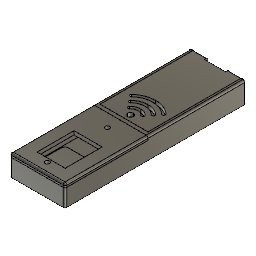
sensor_case (Autodesk Fusion 360 design; units mm, degrees)
Autodesk Fusion 360 part; units mm, degrees
sketch "MainBottom" plane through (0, 0, 0) normal (0, 0, 1) x (1, 0, 0)
  line L0 (0, 0) -> (30, 0)
  line L1 (30, 0) -> (30, 53.3)
  line L2 (30, 53.3) -> (0, 53.3)
  line L3 (0, 53.3) -> (0, 0)
  dimension "d3" = 53.3
  dimension "d4" = 30
  constraint horizontal L0
  constraint vertical L1
  constraint horizontal L2
  constraint vertical L3
  constraint coincident L0.start L3.end
  measures "d3" distance of L0.end L1.end
  measures "d4" distance of L1.end L2.end
extrude "Extrude1" add sketch "MainBottom" along normal blind 2 makes body 1
sketch "MainRight" plane through (30, 0, 0) normal (1, 0, 0) x (0, 1, 0)
  line L0 (0, 0) -> (53.3, 0)
  line L1 (53.3, 0) -> (53.3, 2)
  line L2 (53.3, 2) -> (0, 2)
  line L3 (0, 2) -> (0, 0)
  line L4 (53.3, 2) -> (0, 2)
  line L5 (0, 2) -> (0, 11.5)
  line L6 (0, 11.5) -> (53.3, 11.5)
  line L7 (53.3, 11.5) -> (53.3, 2)
  dimension "d9" = 9.5
  constraint horizontal L4
  constraint vertical L5
  constraint horizontal L6
  constraint vertical L7
  constraint coincident L1.end L2.start
  constraint coincident L2.end L3.start
  measures "d9" distance of L1.end L6.end
extrude "Extrude2" add sketch "MainRight" against normal blind 2 contours L2 L4 L5 L6 L7 bodies 1
sketch "MainLeft" plane through (0, 0, 0) normal (-1, 0, 0) x (0, -1, 0)
  line L0 (-53.3, 0) -> (0, 0)
  line L1 (0, 0) -> (0, 2)
  line L2 (0, 2) -> (-53.3, 2)
  line L3 (-53.3, 2) -> (-53.3, 0)
  line L4 (0, 2) -> (-53.3, 2)
  line L5 (-53.3, 2) -> (-53.3, 11.5)
  line L6 (-53.3, 11.5) -> (0, 11.5)
  line L7 (0, 11.5) -> (0, 2)
  dimension "d12" = 9.5
  constraint horizontal L4
  constraint vertical L5
  constraint horizontal L6
  constraint vertical L7
  constraint coincident L1.end L2.start
  constraint coincident L2.end L3.start
  measures "d12" distance of L1.end L6.end
extrude "Extrude3" add sketch "MainLeft" against normal blind 2 contours L2 L4 L5 L6 L7 bodies 1
sketch "MainFront" plane through (0, 0, 0) normal (0, -1, 0) x (1, 0, 0)
  line L0 (0, 0) -> (30, 0)
  line L1 (30, 0) -> (30, 11.5)
  line L2 (30, 11.5) -> (28, 11.5)
  line L3 (28, 11.5) -> (28, 2)
  line L4 (28, 2) -> (2, 2)
  line L5 (2, 2) -> (2, 11.5)
  line L6 (2, 11.5) -> (0, 11.5)
  line L7 (0, 11.5) -> (0, 0)
  line L8 (2, 2) -> (28, 2)
  line L9 (28, 2) -> (28, 11.5)
  line L10 (28, 11.5) -> (2, 11.5)
  line L11 (2, 11.5) -> (2, 2)
  dimension "d367" = 9.5
  constraint horizontal L8
  constraint vertical L9
  constraint horizontal L10
  constraint vertical L11
  constraint coincident L4.end L5.start
  constraint coincident L3 L2.end
  measures "d367" distance of L3.end L2.end
extrude "Extrude4" add sketch "MainFront" against normal blind 2 contours L3 L4 L5 L8 L9 L10 L11 bodies 1
sketch "MainBack" plane through (0, 53.3, 0) normal (0, 1, 0) x (-1, 0, 0)
  line L0 (-30, 0) -> (0, 0)
  line L1 (0, 0) -> (0, 11.5)
  line L2 (0, 11.5) -> (-2, 11.5)
  line L3 (-2, 11.5) -> (-2, 2)
  line L4 (-2, 2) -> (-28, 2)
  line L5 (-28, 2) -> (-28, 11.5)
  line L6 (-28, 11.5) -> (-30, 11.5)
  line L7 (-30, 11.5) -> (-30, 0)
  line L8 (-28, 2) -> (-2, 2)
  line L9 (-2, 2) -> (-2, 11.5)
  line L10 (-2, 11.5) -> (-28, 11.5)
  line L11 (-28, 11.5) -> (-28, 2)
  constraint horizontal L8
  constraint vertical L9
  constraint horizontal L10
  constraint vertical L11
  constraint coincident L2.end L3.start
  constraint coincident L4.end L5.start
extrude "Extrude5" add sketch "MainBack" against normal blind 2 contours L3 L4 L5 L8 L9 L10 L11 bodies 1
sketch "DeviceSupportBack" plane through (0, 0, 2) normal (0, 0, 1) x (-1, 0, 0)
  line L0 (-28, -51.3) -> (-2, -51.3)
  line L1 (-2, -51.3) -> (-2, -2)
  line L2 (-2, -2) -> (-28, -2)
  line L3 (-28, -2) -> (-28, -51.3)
  line L4 (-28, -51.3) -> (-2, -51.3)
  line L5 (-2, -51.3) -> (-2, -46.3)
  line L6 (-2, -46.3) -> (-28, -46.3)
  line L7 (-28, -46.3) -> (-28, -51.3)
  dimension "d21" = 5
  constraint horizontal L4
  constraint vertical L5
  constraint horizontal L6
  constraint vertical L7
  constraint coincident L1 L5.end
  constraint coincident L0.start L3.end
  measures "d21" distance of L0.start L6.end
sketch "SensorBottom" plane through (0, 0, 0) normal (0, 0, -1) x (1, 0, 0)
  line L0 (0, 0) -> (0, -53.3)
  line L1 (0, -53.3) -> (30, -53.3)
  line L2 (30, -53.3) -> (30, 0)
  line L3 (30, 0) -> (0, 0)
  line L4 (0, 0) -> (30, 0)
  line L5 (30, 0) -> (30, 45)
  line L6 (30, 45) -> (0, 45)
  line L7 (0, 45) -> (0, 0)
  dimension "d144" = 30
  dimension "d145" = 45
  constraint horizontal L4
  constraint vertical L5
  constraint horizontal L6
  constraint vertical L7
  constraint midpoint L3 L4
  measures "d144" distance of L5.end L6.end
  measures "d145" distance of L2.end L5.end
extrude "Extrude17" add sketch "SensorBottom" against normal blind 2 contours L3 L4 L5 L6 L7 bodies 1
extrude "Extrude6" add sketch "DeviceSupportBack" along normal blind 3 contours L0 L1 L3 L4 L5 L6 L7 bodies 1
sketch "DeviceSupportFront" plane through (0, 0, 2) normal (0, 0, 1) x (-1, 0, 0)
  line L0 (-28, -46.3) -> (-2, -46.3)
  line L1 (-2, -46.3) -> (-2, -2)
  line L2 (-2, -2) -> (-28, -2)
  line L3 (-28, -2) -> (-28, -46.3)
  line L4 (-2, -2) -> (-28, -2)
  line L5 (-28, -2) -> (-28, -7)
  line L6 (-28, -7) -> (-2, -7)
  line L7 (-2, -7) -> (-2, -2)
  dimension "d24" = 5
  constraint horizontal L4
  constraint vertical L5
  constraint horizontal L6
  constraint vertical L7
  constraint coincident L3 L5.end
  constraint coincident L1.end L2.start
  measures "d24" distance of L1.end L6.end
extrude "Extrude7" add sketch "DeviceSupportFront" along normal blind 3 contours L1 L2 L3 L4 L5 L6 L7 bodies 1
sketch "DevicePosts" plane through (0, 0, 5) normal (0, 0, 1) x (-1, 0, 0)
  line L0 (-2, -46.3) -> (-28, -46.3)
  circle A0 centre (-25.256, -48.0042) radius 0.95
  line L1 (-2.25, -51) -> (-12.25, -51)
  circle A1 centre (-5.256, -48.0042) radius 0.95
  line L2 (-15.256, -51.0085) -> (-15.256, -2) construction
  line L3 (-15.256, -48.0042) -> (-25.256, -48.0042) construction
  line L4 (-28, -2) -> (-2, -2) construction
  line L5 (-15.256, -26.5042) -> (-15.256, -48.0042) construction
  line L6 (-15.256, -48.0042) -> (-5.256, -48.0042) construction
  line L7 (-15.256, -26.5042) -> (-15.256, -5.0042) construction
  circle A2 centre (-5.256, -5.0042) radius 0.95
  circle A3 centre (-25.256, -5.0042) radius 0.95
  line L8 (-15.256, -5.0042) -> (-5.256, -5.0042) construction
  line L9 (-15.256, -5.0042) -> (-25.256, -5.0042) construction
  line L10 (-28, -46.3) -> (-28, -51.3)
  line L11 (-28, -51.3) -> (-2, -51.3)
  line L12 (-2, -51.3) -> (-2, -46.3)
  dimension "d31" = 1.9
  dimension "d38" = 10
  dimension "d40" = 1.9
  dimension "d59" = 10
  dimension "d60" = 21.5
  dimension "d61" = 10
  dimension "d63" = 1.9
  dimension "d64" = 1.9
  dimension "d65" = 10
  dimension "d67" = 10
  dimension "d68" = 21.5
  constraint vertical L2
  constraint coincident L2 L3.start
  constraint coincident A0.centre L3.end
  constraint perpendicular L2 L3
  constraint coincident L2.end L4
  constraint midpoint L2 L5.start
  constraint parallel L2 L5
  constraint coincident L3.start L5.end
  constraint coincident A1.centre L6.end
  constraint perpendicular L2 L6
  constraint parallel L2 L7
  constraint coincident A2.centre L8.end
  constraint perpendicular L2 L8
  constraint coincident A3.centre L9.end
  constraint perpendicular L7 L9
  measures "d31" diameter of A0
  measures "d38" distance of L1.start L1.end
  measures "d40" diameter of A1
  measures "d59" horizontal distance of L3.start A0.centre
  measures "d60" vertical distance of L5.start L3.start
  measures "d61" distance of L3.start A1.centre
  measures "d63" diameter of A2
  measures "d64" diameter of A3
  measures "d65" horizontal distance of L7.end A2.centre
  measures "d67" horizontal distance of L7.end A3.centre
  measures "d68" distance of L5.start L7.end
extrude "Extrude8" cut sketch "DevicePosts" against normal blind 3 contours A0 | A1 | A2 | A3 bodies 1
sketch "USBPlugOpening" plane through (0, 53.3, 0) normal (0, 1, 0) x (-1, 0, 0)
  line L0 (-30, 0) -> (0, 0)
  line L1 (-15, 7.05) -> (-15, 0) construction
  line L2 (-20.75, 11.175) -> (-9.25, 11.175)
  line L3 (-9.25, 11.175) -> (-9.25, 2.925)
  line L4 (-9.25, 2.925) -> (-20.75, 2.925)
  line L5 (-20.75, 2.925) -> (-20.75, 11.175)
  line L6 (-20.75, 11.175) -> (-9.25, 11.175)
  line L7 (-9.25, 11.175) -> (-9.25, 16.175)
  line L8 (-9.25, 16.175) -> (-20.75, 16.175)
  line L9 (-20.75, 16.175) -> (-20.75, 11.175)
  line L10 (-20.75, 7.05) -> (-9.25, 7.05) construction
  dimension "d392" = 7.05
  dimension "d398" = 11.5
  dimension "d399" = 8.25
  dimension "d400" = 5
  constraint midpoint L0 L1.end
  constraint perpendicular L0 L1
  constraint horizontal L2
  constraint vertical L3
  constraint horizontal L4
  constraint vertical L5
  constraint horizontal L6
  constraint vertical L7
  constraint horizontal L8
  constraint vertical L9
  constraint coincident L2.start L5.end
  constraint coincident L2.end L3.start
  constraint midpoint L5 L10.start
  constraint midpoint L3 L10.end
  constraint midpoint L1.start L10
  measures "d392" distance of L1.start L1.end
  measures "d398" distance of L2.start L2.end
  measures "d399" distance of L2.start L4.end
  measures "d400" distance of L2.start L8.end
ref_plane "WorkPlane1" through (15, 26.65, 5.75) normal (1, 0, 0) x (0, 1, 0)
ref_plane "WorkPlane2" through (15, 26.65, 5.75) normal (0, -1, 0) x (1, 0, 0)
sketch "Lid" plane through (0, 53.3, 0) normal (0, 1, 0) x (-1, 0, 0)
  line L0 (-30, 0) -> (0, 0)
  line L1 (0, 0) -> (0, 11.5)
  line L2 (-30, 11.5) -> (-30, 0)
  line L3 (0, 11.5) -> (-2, 11.5)
  line L4 (-30, 11.5) -> (-28, 11.5) construction
  line L5 (-28, 11.5) -> (-2, 11.5)
  line L6 (-28, 11.5) -> (-29, 9.5)
  line L7 (-29, 9.5) -> (-1, 9.5)
  line L8 (-1, 9.5) -> (-2, 11.5)
  line L9 (-15, 11.5) -> (-15, 9.5) construction
  line L10 (-1, 9.5) -> (0, 9.5) construction
  dimension "d119" = 2
  dimension "d120" = 2
  dimension "d121" = 2
  dimension "d122" = 1
  constraint coincident L1.end L3.start
  constraint perpendicular L1 L3
  constraint coincident L2.start L4.start
  constraint perpendicular L2 L4
  constraint parallel L5 L7
  constraint midpoint L5 L9.start
  constraint midpoint L7 L9.end
  constraint perpendicular L7 L9
  constraint coincident L1 L10.end
  constraint perpendicular L1 L10
  measures "d119" distance of L1.end L3.end
  measures "d120" distance of L2.start L4.end
  measures "d121" vertical distance of L9.start L9.end
  measures "d122" distance of L7.end L10.end
sketch "SensorRIght" plane through (30, 0, 0) normal (1, 0, 0) x (0, 1, 0)
  line L0 (-45, 0) -> (53.3, 0)
  line L1 (0, 11.5) -> (0, 2)
  line L2 (0, 2) -> (-45, 2)
  line L3 (-45, 2) -> (-45, 0)
  line L4 (-45, 2) -> (0, 2)
  line L5 (0, 2) -> (0, 9.5)
  line L6 (0, 9.5) -> (-45, 9.5)
  line L7 (-45, 9.5) -> (-45, 2)
  line L8 (0, 2) -> (0, 11.5)
  line L9 (53.3, 0) -> (53.3, 11.5)
  line L10 (53.3, 11.5) -> (0, 11.5)
  dimension "d155" = 7.5
  constraint horizontal L4
  constraint vertical L5
  constraint horizontal L6
  constraint vertical L7
  constraint coincident L5.end L8
  constraint coincident L2.end L3.start
  measures "d155" distance of L2.end L6.end
extrude "Extrude19" add sketch "SensorRIght" against normal blind 2 contours L1 L2 L4 L5 L6 L7 L8 bodies 1
sketch "SensorLeft" plane through (0, 0, 0) normal (-1, 0, 0) x (0, -1, 0)
  line L0 (-53.3, 0) -> (45, 0)
  line L1 (45, 0) -> (45, 2)
  line L2 (45, 2) -> (0, 2)
  line L3 (0, 2) -> (0, 11.5)
  line L4 (0, 2) -> (45, 2)
  line L5 (45, 2) -> (45, 9.5)
  line L6 (45, 9.5) -> (0, 9.5)
  line L7 (0, 11.5) -> (0, 2)
  line L8 (0, 11.5) -> (-53.3, 11.5)
  line L9 (-53.3, 11.5) -> (-53.3, 0)
  dimension "d372" = 7.5
  constraint horizontal L4
  constraint vertical L5
  constraint horizontal L6
  constraint vertical L7
  constraint coincident L2.end L3.start
  constraint coincident L3.end L7.start
  constraint coincident L1.end L2.start
  constraint coincident L7 L6.end
  measures "d372" distance of L1.end L5.end
extrude "Extrude20" add sketch "SensorLeft" against normal blind 2 contours L2 L3 L4 L5 L6 L7 bodies 1
sketch "SensorFront" plane through (0, -45, 0) normal (0, -1, 0) x (1, 0, 0)
  line L0 (0, 0) -> (30, 0)
  line L1 (30, 0) -> (30, 9.5)
  line L2 (30, 9.5) -> (28, 9.5)
  line L3 (28, 9.5) -> (28, 2)
  line L4 (28, 2) -> (2, 2)
  line L5 (2, 2) -> (2, 9.5)
  line L6 (0, 9.5) -> (0, 0)
  line L7 (2, 2) -> (28, 2)
  line L8 (28, 2) -> (28, 9.5)
  line L9 (28, 9.5) -> (2, 9.5)
  line L10 (2, 9.5) -> (2, 2)
  line L11 (2, 9.5) -> (0, 9.5)
  constraint horizontal L7
  constraint vertical L8
  constraint horizontal L9
  constraint vertical L10
  constraint coincident L2.end L3.start
  constraint coincident L4.end L5.start
extrude "Extrude21" add sketch "SensorFront" against normal blind 2 contours L3 L4 L5 L7 L8 L9 L10 bodies 1
sketch "WireHole" plane through (0, 0, 0) normal (0, -1, 0) x (1, 0, 0)
  line L0 (2, 9.5) -> (2, 2)
  line L1 (2, 2) -> (28, 2)
  line L2 (28, 2) -> (28, 9.5)
  line L3 (11.125, 2) -> (18.875, 2)
  arc A0 (18.875, 2) -> (11.125, 2) centre (15, 2) ccw
  line L4 (30, 11.5) -> (0, 11.5)
  line L5 (0, 9.5) -> (2, 9.5)
  line L6 (30, 9.5) -> (30, 11.5)
  line L7 (28, 9.5) -> (30, 9.5)
  line L8 (0, 11.5) -> (0, 9.5)
  line L9 (15, 2) -> (15, 5.1) construction
  line L10 (17.325, 5.1) -> (12.675, 5.1) construction
  dimension "d162" = 7.75
  dimension "d387" = 3.1
  constraint horizontal L3
  constraint midpoint A0.centre L3
  constraint midpoint L1 A0.centre
  constraint coincident A0.centre L9.start
  constraint perpendicular L3 L9
  constraint horizontal L10
  constraint midpoint L9.end L10
  constraint coincident A0 L10.end
  measures "d162" diameter of A0
  measures "d387" distance of A0.centre L9.end
extrude "Extrude23" cut sketch "WireHole" against normal blind 7 contours L1 L3 A0 bodies 1
sketch "SensorMounts" plane through (0, 0, 2) normal (0, 0, 1) x (-1, 0, 0)
  line L0 (-2, -7) -> (-11.125, -7)
  line L1 (-11.125, -7) -> (-11.125, 0)
  line L2 (-11.125, 0) -> (-2, 0)
  line L3 (-2, 0) -> (-2, 43)
  line L4 (-2, 43) -> (-28, 43)
  line L5 (-28, 43) -> (-28, 0)
  line L6 (-28, 0) -> (-18.875, 0)
  line L7 (-18.875, 0) -> (-18.875, -7)
  line L8 (-18.875, -7) -> (-28, -7)
  line L9 (-28, -7) -> (-28, -46.3)
  line L10 (-28, -46.3) -> (-2, -46.3)
  line L11 (-2, -46.3) -> (-2, -7)
  line L12 (-15, 43) -> (-15, 39.5) construction
  circle A0 centre (-15, 39.5) radius 0.95
  line L13 (-15, 39.5) -> (-15, 37.5) construction
  line L14 (-7.375, 17.5) -> (-22.625, 17.5)
  line L15 (-22.625, 17.5) -> (-22.625, 37.5)
  line L16 (-22.625, 37.5) -> (-7.375, 37.5)
  line L17 (-7.375, 37.5) -> (-7.375, 17.5)
  line L18 (-13, 41.5) -> (-17, 41.5)
  line L19 (-17, 41.5) -> (-17, 37.5)
  line L20 (-17, 37.5) -> (-13, 37.5)
  line L21 (-13, 37.5) -> (-13, 41.5)
  line L22 (-15, 37.5) -> (-15, 41.5) construction
  line L23 (-13, 39.5) -> (-17, 39.5) construction
  circle A1 centre (-15, 39.5) radius 1.2
  line L24 (-22.625, 17.5) -> (-7.375, 17.5)
  line L25 (-7.375, 17.5) -> (-7.375, 22.5)
  line L26 (-7.375, 22.5) -> (-22.625, 22.5)
  line L27 (-22.625, 22.5) -> (-22.625, 17.5)
  circle A2 centre (-15, 7) radius 0.95
  circle A3 centre (-15, 7) radius 1.2
  line L28 (-13, 9) -> (-17, 9)
  line L29 (-17, 9) -> (-17, 5)
  line L30 (-17, 5) -> (-13, 5)
  line L31 (-13, 5) -> (-13, 9)
  line L32 (-15, 5) -> (-15, 9) construction
  line L33 (-13, 7) -> (-17, 7) construction
  line L34 (-15, 0) -> (-15, 7) construction
  line L35 (-2, 0) -> (-28, 0) construction
  dimension "d228" = 3.5
  dimension "d229" = 1.9
  dimension "d230" = 2
  dimension "d231" = 20
  dimension "d232" = 15.25
  dimension "d277" = 4
  dimension "d278" = 4
  dimension "d333" = 2.4
  dimension "d334" = 5
  dimension "d347" = 1.9
  dimension "d348" = 2.4
  dimension "d349" = 4
  dimension "d350" = 4
  dimension "d388" = 7
  constraint midpoint L4 L12.start
  constraint perpendicular L4 L12
  constraint coincident L12.end A0.centre
  constraint parallel L12 L13
  constraint horizontal L14
  constraint vertical L15
  constraint horizontal L16
  constraint vertical L17
  constraint midpoint L13.end L16
  constraint horizontal L18
  constraint vertical L19
  constraint horizontal L20
  constraint vertical L21
  constraint midpoint L20 L13.end
  constraint midpoint L18 L22.end
  constraint midpoint L21 L23.start
  constraint midpoint L19 L23.end
  constraint midpoint L12.end L23
  constraint horizontal L24
  constraint vertical L25
  constraint horizontal L26
  constraint vertical L27
  constraint coincident L17 L25.end
  constraint horizontal L28
  constraint vertical L29
  constraint horizontal L30
  constraint vertical L31
  constraint midpoint L30 L32.start
  constraint midpoint L28 L32.end
  constraint midpoint L31 L33.start
  constraint midpoint L29 L33.end
  constraint midpoint A2.centre L33
  constraint coincident A2.centre A3.centre
  constraint perpendicular L33 L34
  constraint coincident L2.end L3.start
  constraint coincident L5.end L6.start
  constraint midpoint L34.start L35
  measures "d228" distance of L12.start L12.end
  measures "d229" diameter of A0
  measures "d230" distance of L12.end L13.end
  measures "d231" distance of L14.end L15.end
  measures "d232" distance of L14.start L14.end
  measures "d277" distance of L18.start L20.end
  measures "d278" distance of L19.end L20.end
  measures "d333" diameter of A1
  measures "d334" distance of L14.end L26.end
  measures "d347" diameter of A2
  measures "d348" diameter of A3
  measures "d349" distance of L28.start L30.end
  measures "d350" distance of L29.end L30.end
  measures "d388" distance of L34.start A2.centre
extrude "Extrude15" add sketch "Lid" against normal blind 51.3 separate body makes body 2
combine "Combine5" operation cut target body 1 tool bodies 2 keep tools
copy_body "Body->Comp1" bodies 2 removing the originals makes body 3 in component "Case Lid"
extrude "Extrude27" add sketch "SensorMounts" along normal blind 4.9 contours L15 L16 L17 L20 L26 | L16 L18 L19 L20 L21 | A1 bodies 1
extrude "Extrude30" add sketch "SensorMounts" along normal blind 6.4 contours A3 | L28 L29 L30 L31 bodies 1
sketch "LidVents" plane through (0, 0, 11.5) normal (0, 0, 1) x (-1, 0, 0)
  spline S0 degree 3 poles (-15.2286, -9.201) (-14.0919, -9.201) (-12.9552, -8.733) (-12.2197, -7.8637) knots 0 0 0 0 1 1 1 1
  spline S1 degree 3 poles (-12.2197, -7.8637) (-11.551, -7.0613) (-10.3474, -8.1312) (-11.0161, -8.9336) knots 0 0 0 0 1 1 1 1
  spline S2 degree 3 poles (-11.0161, -8.9336) (-12.0859, -10.1372) (-13.6238, -10.8058) (-15.2286, -10.8058) knots 0 0 0 0 1 1 1 1
  spline S3 degree 3 poles (-15.2286, -10.8058) (-16.8334, -10.8058) (-18.3713, -10.1372) (-19.4411, -8.9336) knots 0 0 0 0 1 1 1 1
  spline S4 degree 3 poles (-19.4411, -8.9336) (-20.1098, -8.1312) (-18.9062, -7.0613) (-18.2376, -7.8637) knots 0 0 0 0 1 1 1 1
  spline S5 degree 3 poles (-18.2376, -7.8637) (-17.502, -8.733) (-16.3653, -9.201) (-15.2286, -9.201) knots 0 0 0 0 1 1 1 1
  spline S6 degree 3 poles (-15.2286, -3.5843) (-14.3594, -3.5843) (-13.6238, -4.3199) (-13.6238, -5.1891) knots 0 0 0 0 1 1 1 1
  spline S7 degree 3 poles (-13.6238, -5.1891) (-13.6238, -6.0584) (-14.3594, -6.7939) (-15.2286, -6.7939) knots 0 0 0 0 1 1 1 1
  spline S8 degree 3 poles (-15.2286, -6.7939) (-16.0979, -6.7939) (-16.8334, -6.0584) (-16.8334, -5.1891) knots 0 0 0 0 1 1 1 1
  spline S9 degree 3 poles (-16.8334, -5.1891) (-16.8334, -4.3199) (-16.0979, -3.5843) (-15.2286, -3.5843) knots 0 0 0 0 1 1 1 1
  spline S10 degree 3 poles (-15.2286, -13.213) (-13.0889, -13.213) (-11.1498, -12.4775) (-9.6119, -10.9395) knots 0 0 0 0 1 1 1 1
  spline S11 degree 3 poles (-9.6119, -10.9395) (-8.9433, -10.2709) (-7.6728, -11.2739) (-8.4752, -12.0763) knots 0 0 0 0 1 1 1 1
  spline S12 degree 3 poles (-8.4752, -12.0763) (-10.2806, -13.8816) (-12.6877, -14.8177) (-15.2286, -14.8177) knots 0 0 0 0 1 1 1 1
  spline S13 degree 3 poles (-15.2286, -14.8177) (-17.7695, -14.8177) (-20.1767, -13.8816) (-21.982, -12.0763) knots 0 0 0 0 1 1 1 1
  spline S14 degree 3 poles (-21.982, -12.0763) (-22.7844, -11.2739) (-21.514, -10.2709) (-20.8453, -10.9395) knots 0 0 0 0 1 1 1 1
  spline S15 degree 3 poles (-20.8453, -10.9395) (-19.3074, -12.4775) (-17.3683, -13.213) (-15.2286, -13.213) knots 0 0 0 0 1 1 1 1
  spline S16 degree 3 poles (-15.2286, -17.2249) (-12.1528, -17.2249) (-9.2776, -16.0882) (-7.071, -14.0154) knots 0 0 0 0 1 1 1 1
  spline S17 degree 3 poles (-7.071, -14.0154) (-6.2686, -13.2798) (-5.1319, -14.4166) (-5.9343, -15.1521) knots 0 0 0 0 1 1 1 1
  spline S18 degree 3 poles (-5.9343, -15.1521) (-8.5421, -17.5592) (-11.7516, -18.8297) (-15.2286, -18.8297) knots 0 0 0 0 1 1 1 1
  spline S19 degree 3 poles (-15.2286, -18.8297) (-18.7056, -18.8297) (-21.9152, -17.5592) (-24.5229, -15.1521) knots 0 0 0 0 1 1 1 1
  spline S20 degree 3 poles (-24.5229, -15.1521) (-25.3253, -14.4166) (-24.1886, -13.2798) (-23.3862, -14.0154) knots 0 0 0 0 1 1 1 1
  spline S21 degree 3 poles (-23.3862, -14.0154) (-21.1796, -16.0882) (-18.3044, -17.2249) (-15.2286, -17.2249) knots 0 0 0 0 1 1 1 1
extrude "Extrude1'" cut sketch "LidVents" against normal blind 2 bodies 3 in component "Case Lid"
extrude "Extrude2'" cut sketch "SensorMounts" along normal blind 9.5 contours A0 | L15 L16 L17 L20 L26 | A1 | A2 | A3 bodies 3 in component "Case Lid"
sketch "SensorLid" plane through (0, 0, 9.5) normal (0, 0, 1) x (-1, 0, 0)
  line L0 (-30, 45) -> (-30, 0)
  line L1 (0, 0) -> (0, 45)
  line L2 (0, 45) -> (-30, 45)
  line L3 (0, 0) -> (-30, 0)
  constraint coincident L1.start L3.start
  constraint coincident L0.end L3.end
extrude "Extrude1''" add sketch "SensorLid" along normal blind 2 separate body makes body 4 in component "SensorLid"
extrude "Extrude2''" cut sketch "SensorMounts" along normal blind 9.5 contours A0 | L14 L15 L17 L24 L25 L26 L27 | L15 L16 L17 L20 L26 | A1 | A2 | A3 bodies 4 in component "SensorLid"
fillet "Fillet12" radius 1 4 edges at (30, -45, 4.75) (0, -45, 4.75) (0, 53.3, 5.75) (30, 53.3, 5.75) on bodies 1
fillet "Fillet1" radius 1 2 edges at (30, -45, 10.5) (0, -45, 10.5) on bodies 4 in component "SensorLid"
fillet "Fillet4" radius 1 1 edges at (15, 53.3, 11.5) on bodies 3 in component "Case Lid"
fillet "Fillet13" radius 1 6 edges at (30, 26.15, 11.5) (29.7071, 53.0071, 11.5) (28.5, 53.3, 11.5) (1.5, 53.3, 11.5) (0.2929, 53.0071, 11.5) (0, 26.15, 11.5) on bodies 1
fillet "Fillet2" radius 1 5 edges at (0, -22, 11.5) (0.2929, -44.7071, 11.5) (15, -45, 11.5) (29.7071, -44.7071, 11.5) (30, -22, 11.5) on bodies 4 in component "SensorLid"
extrude "Extrude31" cut sketch "USBPlugOpening" against normal blind 2 bodies 1
extrude "Extrude4'" cut sketch "USBPlugOpening" against normal blind 2 bodies 3 in component "Case Lid"
fillet "Fillet15" radius 2 10 edges at (22.625, -37.5, 4.45) (22.625, -22.5, 4.45) (17, -41.5, 4.45) (7.375, -37.5, 4.45) (7.375, -22.5, 4.45) (13, -41.5, 4.45) (17, -9, 5.2) (17, -5, 5.2) (13, -9, 5.2) (13, -5, 5.2) on bodies 1
component "Case Lid" placed x (1, 0, 0) y (0, 1, 0) z (0, 0, 1) at (0, 0, 0)
component "SensorLid" placed x (1, 0, 0) y (0, 1, 0) z (0, 0, 1) at (0, 0, 0)
equation "MainBaseLength = 49.30 mm + ( MaterialThickness * 2 )"
equation "MainBaseWidth = 26 mm + ( MaterialThickness * 2 )"
equation "d3 = MainBaseLength"
equation "d4 = MainBaseWidth"
equation "MaterialThickness = 2 mm"
equation "d6 = MaterialThickness"
equation "MainBaseHeight = SensorWallsHeight + MaterialThickness"
equation "d9 = MainBaseHeight"
equation "d10 = -MaterialThickness"
equation "d12 = MainBaseHeight"
equation "d13 = -MaterialThickness"
equation "d15 = -MaterialThickness"
equation "d17 = -MaterialThickness"
equation "DeviceSupportHeight = 3 mm"
equation "DeviceSupportLength = 5 mm"
equation "d21 = DeviceSupportLength"
equation "d22 = DeviceSupportHeight"
equation "d24 = DeviceSupportLength"
equation "d25 = DeviceSupportHeight"
equation "EdgeFillet = 1 mm"
equation "d31 = DeviceScrewHoleDiameter"
equation "d32 = -DeviceSupportHeight"
equation "DevicePostYFromCenter = 21.5 mm"
equation "DevicePostXFromCenter = 10 mm"
equation "DeviceScrewHoleDiameter = 1.9 mm"
equation "d38 = DevicePostXFromCenter"
equation "d40 = DeviceScrewHoleDiameter"
equation "InnerEdgeFillet = 2 mm"
equation "USBPlugOpeningWidth = 11.5 mm"
equation "USBPlugOpeningHeight = 8.25 mm"
equation "ConnectorOpeningFillet = 0.5 mm"
equation "d59 = DevicePostXFromCenter"
equation "d60 = DevicePostYFromCenter"
equation "d61 = DevicePostXFromCenter"
equation "d63 = DeviceScrewHoleDiameter"
equation "d64 = DeviceScrewHoleDiameter"
equation "d65 = DevicePostXFromCenter"
equation "d67 = DevicePostXFromCenter"
equation "d68 = DevicePostYFromCenter"
equation "TopFillet = 1 mm"
equation "d119 = MaterialThickness"
equation "d120 = MaterialThickness"
equation "d121 = MaterialThickness"
equation "d122 = MaterialThickness / 2"
equation "d123 = -MainBaseLength + MaterialThickness"
equation "SensorBaseLength = 45 mm"
equation "SensorBaseWidth = MainBaseWidth"
equation "d144 = SensorBaseWidth"
equation "d145 = SensorBaseLength"
equation "d146 = -MaterialThickness"
equation "SensorLength = 20 mm"
equation "SensorWidth = 15.25 mm"
equation "SensorWallsHeight = 7.5 mm"
equation "d155 = SensorWallsHeight"
equation "d156 = -MaterialThickness"
equation "d158 = -MaterialThickness"
equation "d160 = -MaterialThickness"
equation "d162 = MainBaseWireHoleDiameter"
equation "MainBaseWireHoleDiameter = ( 3.25 mm * 2 ) + 1.25 mm"
equation "d166 = -DeviceSupportLength - MaterialThickness"
equation "SensorScrewHoleDimension = 1.9 mm"
equation "SensorScrewHoleIndent = 3.5 mm"
equation "SensorScrewHoleToSensorTop = 2 mm"
equation "d228 = SensorScrewHoleIndent"
equation "d229 = SensorScrewHoleDimension"
equation "d230 = SensorScrewHoleToSensorTop"
equation "d231 = SensorLength"
equation "d232 = SensorWidth"
equation "SensorBaseThickness = 1.6 mm"
equation "SensorConnectorGapWidth = 10 mm"
equation "SensorConnectorGapLength = 1 mm"
equation "d277 = d230 * 2"
equation "d278 = d277"
equation "d279 = SensorPlatformHeight"
equation "d305 = -MaterialThickness"
equation "d333 = d229 + 0.5 mm"
equation "SensorPlatformHeight = SensorWallsHeight - SensorBaseThickness - 1 mm"
equation "SensorLidPlatformSpacer = SensorWallsHeight - SensorPlatformHeight - SensorBaseThickness"
equation "d347 = d229"
equation "d348 = d333"
equation "d349 = d277"
equation "d350 = d278"
equation "d351 = SensorPlatformHeight + SensorBaseThickness - 0.1 mm"
equation "d366 = SensorBaseLength + 10 mm"
equation "d367 = MainBaseHeight"
equation "d368 = SensorWallsHeight + MaterialThickness"
equation "d372 = SensorWallsHeight"
equation "d373 = MaterialThickness"
equation "d375 = SensorWallsHeight + MaterialThickness"
equation "d377 = EdgeFillet"
equation "d378 = EdgeFillet"
equation "d379 = TopFillet"
equation "d380 = TopFillet"
equation "d381 = TopFillet"
equation "USBPlugLidFillerHeight = 0.25 mm"
equation "d388 = SensorLidSecondaryScrewIndent"
equation "SensorLidSecondaryScrewIndent = 7 mm"
equation "d392 = DeviceSupportHeight + MaterialThickness + 2.05 mm"
equation "d393 = -MaterialThickness"
equation "d395 = -MaterialThickness"
equation "d398 = USBPlugOpeningWidth"
equation "d399 = USBPlugOpeningHeight"
equation "d402 = InnerEdgeFillet"
named bodies: "Case Bottom", "Case Lid"
